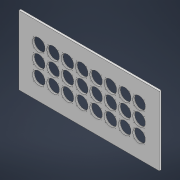
# Autodesk Inventor part: Board
Saved by Autodesk Inventor 2021 (Build 250183000, 183)
## iProperties
Created: 2021-03-25
Part Number: Board
Material: Generic
Document SubType Name: Modeling
Designer: allen
Density: 1 g/cm^3
Appearance: Default
Author: allen
Autodesk Inventor part; units mm, degrees
sketch "Sketch1" plane through (0, 0, 0) normal (0, 0, 1) x (1, 0, 0)
  line L0 (0, 0) -> (1030, 0)
  line L1 (1030, 0) -> (1030, 505)
  line L2 (1030, 505) -> (0, 505)
  line L3 (0, 505) -> (0, 0)
  dimension "d0" = 1030
  dimension "d1" = 505
  constraints: 8 end point, 2 parallel, 1 horizontal, 1 perpendicular
  measures "d0" distance of L0.start L0.end
  measures "d1" distance of L2.end L0.start
extrude "Extrusion1" add sketch "Sketch1" along normal blind 15
sketch "Sketch2" plane through (0, 0, 15) normal (0, 0, 1) x (1, 0, 0)
  line L0 (1030, 505) -> (0, 505) projected
  line L1 (0, 505) -> (0, 0) projected
  point P0 (147, 358)
  dimension "d4" = 147
  dimension "d5" = 147
  measures "d4" distance from line of L0 point (147, 358)
  measures "d5" distance from line of L1 point (147, 358)
hole "Hole1" at (147, 358, 15) direction (0, 0, -1) diameter 92 end through all
sketch "Sketch3" plane through (0, 0, 15) normal (0, 0, 1) x (1, 0, 0)
  circle A0 centre (147, 358) radius 46 projected
  circle A1 centre (147, 358) radius 52.5
  line L0 (147, 358) -> (101, 358)
  line L1 (147, 358) -> (109.8769, 395.1231)
  point P0 (0, 0)
  point P1 (109.8769, 320.8769)
  point P2 (184.1231, 320.8769)
  point P3 (184.1231, 395.1231)
  dimension "d40" = 105
  dimension "d41" = 45
  dimension "d44" = 360
  constraints: 4 end point, 2 coincident, 1 horizontal, 1 horizontal alignment, 9 other
  measures "d41" angle of L0 L1
hole "Hole2" at (184.1231, 395.1231, 15) at (184.1231, 320.8769, 15) at (109.8769, 320.8769, 15) at (109.8769, 395.1231, 15) direction (0, 0, -1) diameter 2.8 depth 8 tip angle 118
pattern_linear "Rectangular Pattern1" count 8 spacing 105 along (1, 0, 0) count 3 spacing 105 along (0, -1, 0) of "Hole1", "Hole2"
sketch "Sketch4" plane through (0, 0, 15) normal (0, 0, 1) x (1, 0, 0)
  line L0 (1030, 505) -> (0, 505) projected
  line L1 (0, 505) -> (0, 0) projected
  line L2 (1030, 0) -> (1030, 505) projected
  line L3 (0, 0) -> (1030, 0) projected
  line L4 (67.5, 68) -> (67.5, 437)
  line L5 (67.5, 437) -> (962.5, 437)
  point P0 (962.5, 68)
  point P1 (67.5, 252.5)
  point P2 (0, 252.5)
  point P3 (515, 437)
  point P4 (515, 505)
  dimension "d39" = 369
  dimension "d46" = 895
  constraints: 4 end point, 4 midpoint, 3 horizontal alignment, 2 coincident, 2 vertical alignment, 1 horizontal, 1 perpendicular
  measures "d39" distance of L4.start L4.end
  measures "d46" distance from line of L5.end L4
hole "Hole3" [suppressed]
ref_plane "Work Plane1" through (0, 252.5, 0) normal (0, 1, 0) x (1, 0, 0)
ref_plane "Work Plane2" through (515, 0, 0) normal (1, 0, 0) x (0, 0, -1)
ref_plane "Work Plane3" through (0, 68, 0) normal (0, -1, 0) x (1, 0, 0)
equation "\"d5\" = d4"
body "Solid1"
